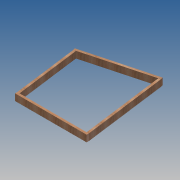
# Autodesk Inventor part: panelCflat
Saved by Autodesk Inventor 2014 SP1 (Build 180222100, 222)
## iProperties
Created: 2015-02-12
Part Number: panelCflat
Material: Wood (Birch)
Document SubType Name: Modeling
Designer: Dave
Density: 0.55 g/cm^3
Appearance: Birch - Natural Polished
Mass: 11947.1 g
Surface Area: 15243.5 cm^2
Volume: 21722 cm^3
Author: Dave
Autodesk Inventor part; units mm, degrees
ref_plane "YZ Plane" through (0, 0, 0) normal (1, 0, 0) x (0, 1, 0)
ref_plane "XZ Plane" through (0, 0, 0) normal (0, 1, 0) x (-1, 0, 0)
ref_plane "XY Plane" through (0, 0, 0) normal (0, 0, 1) x (1, 0, 0)
sketch "Sketch1" plane through (0, 0, 0) normal (0, 1, 0) x (-1, 0, 0)
  line L0 (0, 0) -> (-12922.0343, 0) construction
  line L1 (0, 0) -> (-12360.1465, -3311.8913) construction
  line L2 (0, 0) -> (13412.8311, 0) construction
  line L3 (-4192.3928, 50) -> (-5417.1104, 50)
  line L4 (-4036.5995, -1133.3674) -> (-5219.5859, -1450.3476)
  line L5 (-5417.1104, 12) -> (-5229.4211, -1413.6425)
  line L6 (-4041.5281, -1095.9314) -> (-4187.39, 12)
  line L7 (0, 0) -> (-4114.4962, -541.6837) construction
  line L8 (0, 0) -> (4150, 0) construction
  line L9 (-5378.7825, 12) -> (-4225.7179, 12)
  line L10 (-4225.7179, 12) -> (-4078.6242, -1105.2874)
  line L11 (-4078.6242, -1105.2874) -> (-5192.3991, -1403.7225)
  line L12 (-5192.3991, -1403.7225) -> (-5378.7825, 12)
  line L13 (-5378.7825, 12) -> (-5445.5914, 12) construction
  line L14 (-5417.1104, 12) -> (-5417.1104, 50)
  line L15 (-4225.7179, 12) -> (-4187.39, 12) construction
  line L16 (-4187.39, 12) -> (-4187.39, 50)
  line L17 (-4187.39, 50) -> (-4192.3928, 50)
  line L18 (-4076.4449, -1105.2874) -> (-4041.5281, -1095.9314) construction
  line L19 (-4041.5281, -1095.9314) -> (-4031.8389, -1132.0918)
  line L20 (-4031.8389, -1132.0918) -> (-4036.5995, -1133.3674)
  line L21 (-5192.3991, -1403.7225) -> (-5229.4211, -1413.6425) construction
  line L22 (-5229.4211, -1413.6425) -> (-5219.5859, -1450.3476)
  dimension "d0" = 165
  dimension "d3" = 50
  dimension "d4" = 50
  dimension "d6" = 4150
  dimension "d7" = 172.5
  dimension "d10" = 38
  constraints: 46 end point, 7 perpendicular, 6 parallel, 3 horizontal, 3 point on line, 2 collinear, 1 equal length
  measures "d0" angle of L1 L2
  measures "d3" distance between parallel lines of L3 L0
  measures "d4" distance between parallel lines of L1 L4
  measures "d6" distance of L7.end L0.start
  measures "d7" angle of L7 L8
  measures "d10" distance between parallel lines of L9 L3
extrude "Extrusion2" add sketch "Sketch1" along normal blind 114
sketch "Sketch2" plane through (0, 114, 0) normal (0, 1, 0) x (1, 0, 0)
  line L0 (4225.7179, -12) -> (4078.6242, 1105.2874) projected
  line L1 (4041.5281, 1095.9314) -> (4187.39, -12) projected
  line L2 (4187.39, -12) -> (4187.39, -50) projected
  line L3 (4078.6242, 1105.2874) -> (4041.5281, 1095.9314)
  line L4 (4225.7179, -12) -> (4187.39, -12)
  point P0 (0, 0)
  constraints: 4 end point, 1 perpendicular
extrude "Extrusion3" cut sketch "Sketch2" against normal blind 1
sketch "Sketch3" plane through (0, 114, 0) normal (0, 1, 0) x (1, 0, 0)
  line L0 (5192.3991, 1403.7225) -> (5378.7825, -12) projected
  line L1 (5417.1104, -50) -> (5417.1104, -12) projected
  line L2 (5417.1104, -12) -> (5229.4211, 1413.6425) projected
  line L3 (4031.8389, 1132.0918) -> (4041.5281, 1095.9314) projected
  line L4 (5192.3991, 1403.7225) -> (5229.4211, 1413.6425)
  line L5 (5378.7825, -12) -> (5417.1104, -12)
  point P0 (0, 0)
  constraints: 4 end point, 2 perpendicular
extrude "Extrusion4" cut sketch "Sketch3" against normal blind 1
body "Solid2"
